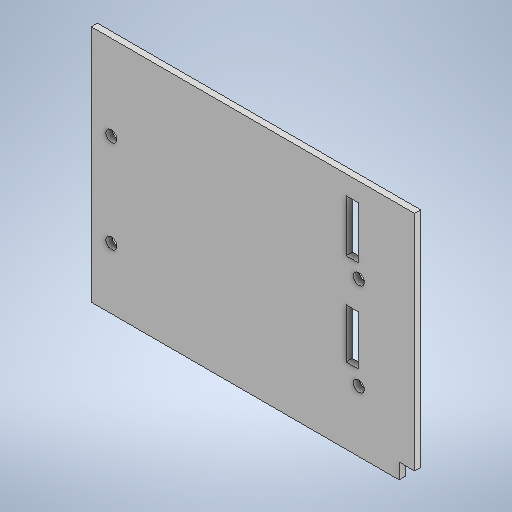
# Autodesk Inventor part: Baseplate_for_PCBs_v2_section_topRight
Saved by Autodesk Inventor 2025.1 (Build 291241000, 241)
## iProperties
Created: 2025-04-15
Part Number: Baseplate_for_PCBs_v2_section_topRight
Material: Generic
Document SubType Name: Modeling
Designer: edward.horrocks
Density: 1 g/cm^3
Appearance: Default
Author: edward.horrocks
Autodesk Inventor part; units mm, degrees
ref_plane "YZ Plane" through (0, 0, 0) normal (1, 0, 0) x (0, 1, 0)
ref_plane "XZ Plane" through (0, 0, 0) normal (0, 1, 0) x (-1, 0, 0)
ref_plane "XY Plane" through (0, 0, 0) normal (0, 0, 1) x (1, 0, 0)
sketch "Sketch2" plane through (0, 0, 0) normal (0, 0, 1) x (1, 0, 0)
  line L0 (-104.5, 104.5) -> (104.5, 104.5)
  line L1 (104.5, 104.5) -> (104.5, -104.5)
  line L2 (104.5, -104.5) -> (-104.5, -104.5)
  line L3 (-104.5, -104.5) -> (-104.5, 104.5)
  line L4 (-104.5, 104.5) -> (104.5, -104.5) construction
  line L5 (104.5, 104.5) -> (-104.5, -104.5) construction
  line L6 (-104.5, 104.5) -> (-99.5, 104.5)
  line L7 (-99.5, 104.5) -> (-99.5, 99.5)
  line L8 (-99.5, 99.5) -> (-104.5, 99.5)
  line L9 (-104.5, 99.5) -> (-104.5, 104.5)
  line L10 (104.5, 104.5) -> (99.5, 104.5)
  line L11 (99.5, 104.5) -> (99.5, 99.5)
  line L12 (99.5, 99.5) -> (104.5, 99.5)
  line L13 (104.5, 99.5) -> (104.5, 104.5)
  line L14 (104.5, -104.5) -> (99.5, -104.5)
  line L15 (99.5, -104.5) -> (99.5, -99.5)
  line L16 (99.5, -99.5) -> (104.5, -99.5)
  line L17 (104.5, -99.5) -> (104.5, -104.5)
  line L18 (-104.5, -104.5) -> (-99.5, -104.5)
  line L19 (-99.5, -104.5) -> (-99.5, -99.5)
  line L20 (-99.5, -99.5) -> (-104.5, -99.5)
  line L21 (-104.5, -99.5) -> (-104.5, -104.5)
  line L22 (-90, 90) -> (90, -90) construction
  line L23 (90, 90) -> (-90, -90) construction
  point P0 (0, 0)
  point P1 (-104.5, -99.5)
  point P2 (99.5, -104.5)
  point P3 (99.5, 104.5)
  point P4 (-99.5, 104.5)
  point P5 (-104.5, 99.5)
  dimension "d0" = 209
  dimension "d1" = 209
  dimension "d2" = 5
  dimension "d3" = 5
  dimension "d4" = 5
  dimension "d5" = 5
  dimension "d6" = 5
  dimension "d7" = 5
  dimension "d8" = 5
  dimension "d9" = 5
  constraints: 48 end point, 10 parallel, 5 horizontal, 5 perpendicular, 4 midpoint
  measures "d0" distance of L1.end L2.end
  measures "d1" distance of L0.end L1.end
  measures "d2" distance of L7.end L8.end
  measures "d3" distance of L6.end L7.end
  measures "d4" distance of L12.end L11.end
  measures "d5" distance of L11.end L10.end
  measures "d6" distance of L15.end L16.end
  measures "d7" distance of L14.end L15.end
  measures "d8" distance of L20.end L19.end
  measures "d9" distance of L19.end L18.end
extrude "Extrusion1" add sketch "Sketch2" along normal blind 2 contours L0 L11 L12 L1 L16 L15 L2 L19 L20 L3 L8 L7
sketch "Sketch3" plane through (0, 0, 2) normal (0, 0, 1) x (1, 0, 0)
  circle A0 centre (-85, 86.25) radius 1.825
  point P0 (0, 0)
  dimension "d18" = 3.65
  constraints: 1 centre point
  measures "d18" diameter of A0
hole "Hole1" at (-85, 86.25, 2) direction (0, 0, -1) diameter 3.6 depth 10
pattern_linear "Rectangular Pattern1" count 2 spacing 80 along (1, 0, 0) count 6 spacing 30 along (0, -1, 0) of "Hole1"
sketch "Sketch4" plane through (0, 0, 2) normal (0, 0, 1) x (1, 0, 0)
  circle A0 centre (6.5, 65.25) radius 1.8
  line L0 (99.5, 104.5) -> (-99.5, 104.5) projected
  point P0 (0, 0)
  dimension "d33" = 3.6
  dimension "d47" = 39.25
  constraints: 1 centre point
  measures "d33" diameter of A0
  measures "d47" distance from line of L0 A0.centre
hole "Hole2" at (6.5, 65.25, 2) direction (0, 0, -1) diameter 3.6 depth 10
pattern_linear "Rectangular Pattern2" count 2 spacing 80 along (1, 0, 0) count 6 spacing 30 along (0, -1, 0) of "Hole2"
sketch "Sketch5" plane through (0, 0, 2) normal (0, 0, 1) x (1, 0, 0)
  line L0 (-84.848, 81.55) -> (-80.848, 81.55)
  line L1 (-80.848, 81.55) -> (-80.848, 65.55)
  line L2 (-80.848, 65.55) -> (-84.848, 65.55)
  line L3 (-84.848, 65.55) -> (-84.848, 81.55)
  line L4 (-84.848, 51.79) -> (-80.848, 51.79)
  line L5 (-80.848, 51.79) -> (-80.848, 35)
  line L6 (-80.848, 35) -> (-84.848, 35)
  line L7 (-84.848, 35) -> (-84.848, 51.79)
  point P0 (0, 0)
  dimension "d51" = 4
  dimension "d52" = 16
  dimension "d65" = 4
  dimension "d66" = 16.79
  constraints: 16 end point, 4 parallel, 2 horizontal, 2 perpendicular
  measures "d51" distance of L1.end L2.end
  measures "d52" distance of L0.end L1.end
  measures "d65" distance of L5.end L6.end
  measures "d66" distance of L4.end L5.end
extrude "Extrusion2" cut sketch "Sketch5" against normal blind 10
pattern_linear "Rectangular Pattern5" count 3 spacing 60 along (0, -1, 0) of "Extrusion2"
sketch "Sketch7" plane through (0, 0, 2) normal (0, 0, 1) x (1, 0, 0)
  line L0 (86.348, -80.05) -> (82.348, -80.05)
  line L1 (82.348, -80.05) -> (82.348, -64.05)
  line L2 (82.348, -64.05) -> (86.348, -64.05)
  line L3 (86.348, -64.05) -> (86.348, -80.05)
  line L4 (86.348, -50.29) -> (82.348, -50.29)
  line L5 (82.348, -50.29) -> (82.348, -33.5)
  line L6 (82.348, -33.5) -> (86.348, -33.5)
  line L7 (86.348, -33.5) -> (86.348, -50.29)
  point P0 (0, 0)
  dimension "d70" = 4
  dimension "d71" = 16
  dimension "d72" = 4
  dimension "d73" = 16.79
  constraints: 16 end point, 4 parallel, 2 horizontal, 2 perpendicular
  measures "d70" distance of L1.end L2.end
  measures "d71" distance of L0.end L1.end
  measures "d72" distance of L5.end L6.end
  measures "d73" distance of L4.end L5.end
extrude "Extrusion4" cut sketch "Sketch7" against normal blind 10
pattern_linear "Rectangular Pattern6" count 3 spacing 60 along (0, 1, 0) of "Extrusion4"
sketch "Sketch8" plane through (0, 0, 2) normal (0, 0, 1) x (1, 0, 0)
  line L0 (105.3231, -105.4618) -> (0, -105.4618)
  line L1 (0, -105.4618) -> (0, -27.3986)
  line L2 (0, -27.3986) -> (105.3231, -27.3986)
  line L3 (105.3231, -27.3986) -> (105.3231, -105.4618)
  point P0 (0, 0)
  constraints: 8 end point, 2 parallel, 1 horizontal, 1 perpendicular
extrude "Extrusion5" cut sketch "Sketch8" against normal blind 10 keep common part
body "Solid1"
